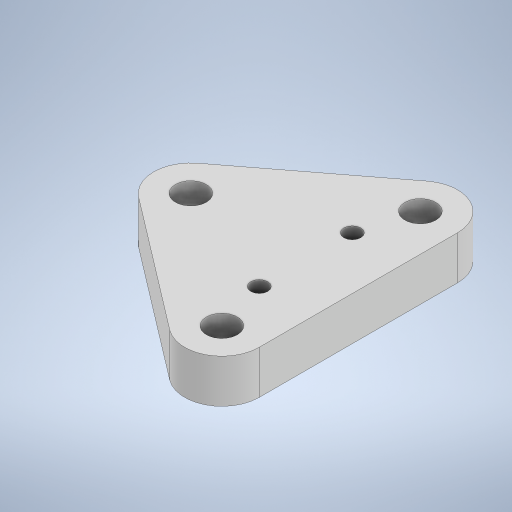
# Autodesk Inventor part: base_obj4
Saved by Autodesk Inventor 2023.2 (Build 272271030, 271C)
## iProperties
Created: 2023-02-25
Part Number: base_obj4
Material: Generic
Document SubType Name: Modeling
Designer: Cris Pat
Density: 1 g/cm^3
Appearance: Default
Author: Cris Pat
Autodesk Inventor part; units mm, degrees
ref_plane "YZ Plane" through (0, 0, 0) normal (1, 0, 0) x (0, 1, 0)
ref_plane "XZ Plane" through (0, 0, 0) normal (0, 1, 0) x (-1, 0, 0)
ref_plane "XY Plane" through (0, 0, 0) normal (0, 0, 1) x (1, 0, 0)
sketch "Sketch1" plane through (0, 0, 0) normal (0, 1, 0) x (-1, 0, 0)
  circle A0 centre (0, 32) radius 5
  circle A1 centre (0, -32) radius 5
  circle A2 centre (42, 0) radius 5
  circle A3 centre (0, -32) radius 12 construction
  circle A4 centre (42, 0) radius 12 construction
  circle A5 centre (0, 32) radius 12 construction
  line L0 (-12, -32) -> (-12, 32)
  line L1 (7.2725, 41.5452) -> (49.2725, 9.5452)
  line L2 (49.2725, -9.5452) -> (7.2725, -41.5452)
  arc A6 (7.2725, 41.5452) -> (-12, 32) centre (0, 32) ccw
  arc A7 (-12, -32) -> (7.2725, -41.5452) centre (0, -32) ccw
  arc A8 (49.2725, -9.5452) -> (49.2725, 9.5452) centre (42, 0) ccw
  point P0 (0, 0)
  dimension "d0" = 10
  dimension "d1" = 64
  dimension "d2" = 32
  dimension "d3" = 24
  dimension "d4" = 42
  constraints: 12 point on circle, 10 tangent, 9 centre point, 6 end point, 5 equal radius, 3 coincident, 2 vertical alignment, 1 horizontal alignment
  measures "d0" diameter of A0
  measures "d1" distance of A1.centre A0.centre
  measures "d2" vertical distance of A0.centre A2.centre
  measures "d3" diameter of A3
  measures "d4" horizontal distance of A1.centre A2.centre
extrude "Extrusion1" add sketch "Sketch1" along normal blind 14
sketch "Sketch3" plane through (0, 0, 0) normal (0, -1, 0) x (1, 0, 0)
  line L0 (-49.2725, 9.5452) -> (-7.2725, 41.5452) construction
  arc A0 (-49.2725, 9.5452) -> (-49.2725, -9.5452) centre (-42, 0) ccw construction
  line L1 (-7.2725, -41.5452) -> (-49.2725, -9.5452) construction
  arc A1 (-7.2725, -41.5452) -> (12, -32) centre (0, -32) ccw construction
  line L2 (12, 32) -> (12, -32) construction
  arc A2 (12, 32) -> (-7.2725, 41.5452) centre (0, 32) ccw construction
  circle A3 centre (-42, 0) radius 5 construction
  circle A4 centre (0, -32) radius 5 construction
  circle A5 centre (0, 32) radius 5 construction
  line L3 (12, 32) -> (12, -32) construction
  line L4 (12, 0) -> (-42, 0) construction
  line L5 (12, 20) -> (2, 20) construction
  line L6 (2, 20) -> (2, -20) construction
  line L7 (2, -20) -> (12, -20) construction
  line L8 (12, -20) -> (12, 20) construction
  circle A6 centre (-4.95, -15) radius 2.75
  circle A7 centre (-4.95, 15) radius 2.75
  point P0 (0, 0)
  point P1 (7, -20)
  dimension "d7" = 10
  dimension "d8" = 40
  dimension "d9" = 5.5
  dimension "d10" = 5
  dimension "d11" = 6.95
  constraints: 10 end point, 5 midpoint, 3 coincident, 2 centre point, 2 parallel, 1 horizontal, 1 perpendicular, 1 symmetric about line, 1 other
  measures "d7" distance of L7.end L6.end
  measures "d8" distance of L6.end L5.end
  measures "d9" diameter of A6
  measures "d10" vertical distance of A6.centre point (7, -20)
  measures "d11" distance from line of A6.centre L6
extrude "Extrusion2" cut sketch "Sketch3" against normal through all
equation "\"d2\" = 0.5 * d1"
body "Solid1"
